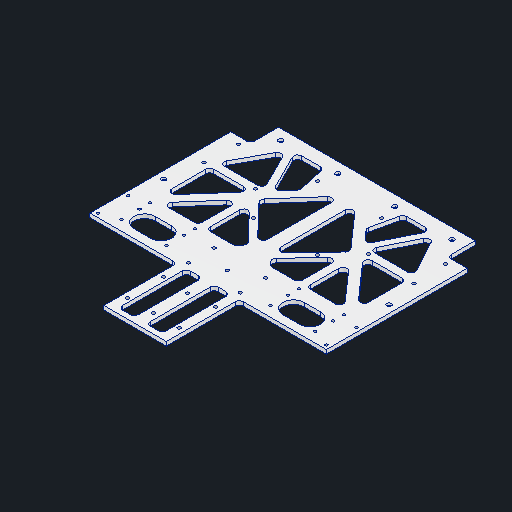
# Autodesk Inventor part: base
Saved by Autodesk Inventor 2023 (Build 270158000, 158)
## iProperties
Created: 2024-04-10
Part Number: base
Material: Aluminum 6061
Document SubType Name: Modeling
Designer: szymo
Density: 2.7 g/cm^3
Appearance: Aluminum - Flat
Mass: 125.073 g
Surface Area: 388.104 cm^2
Volume: 46.3232 cm^3
Author: szymo
Autodesk Inventor part; units mm, degrees
ref_plane "YZ Plane" through (0, 0, 0) normal (1, 0, 0) x (0, 1, 0)
ref_plane "XZ Plane" through (0, 0, 0) normal (0, 1, 0) x (-1, 0, 0)
ref_plane "XY Plane" through (0, 0, 0) normal (0, 0, 1) x (1, 0, 0)
sketch "Sketch2" plane through (0, 0, 0) normal (0, 1, 0) x (-1, 0, 0)
  line L0 (-89, 99) -> (89, 99)
  line L1 (89, 99) -> (89, -99)
  line L2 (89, -99) -> (-89, -99)
  line L3 (-89, -99) -> (-89, 99)
  line L4 (-89, 99) -> (89, -99) construction
  line L5 (89, 99) -> (-89, -99) construction
  line L6 (-89, 99) -> (89, 99)
  line L7 (89, 99) -> (89, -85)
  line L8 (89, -85) -> (-89, -85)
  line L9 (-89, -85) -> (-89, 99)
  line L10 (-4.5, 99) -> (-89, 99)
  line L11 (-89, 99) -> (-89, 42)
  line L12 (-89, 42) -> (-4.5, 42)
  line L13 (-4.5, 42) -> (-4.5, 99)
  line L14 (4.5, 99) -> (89, 99)
  line L15 (89, 99) -> (89, 42)
  line L16 (89, 42) -> (4.5, 42)
  line L17 (4.5, 42) -> (4.5, 99)
  line L18 (22.5, 77.5) -> (22.5, 66.5) projected
  line L19 (16.5, 66.5) -> (16.5, 77.5) projected
  line L20 (-22.5, 66.5) -> (-22.5, 77.5) projected
  line L21 (-16.5, 77.5) -> (-16.5, 66.5) projected
  line L22 (-23.5, 99) -> (-16.5, 99)
  line L23 (-16.5, 99) -> (-16.5, 42)
  line L24 (-16.5, 42) -> (-23.5, 42)
  line L25 (-23.5, 42) -> (-23.5, 99)
  line L26 (16.5, 99) -> (23.5, 99)
  line L27 (23.5, 99) -> (23.5, 42)
  line L28 (23.5, 42) -> (16.5, 42)
  line L29 (16.5, 42) -> (16.5, 99)
  line L30 (-89, 99) -> (89, 99)
  line L31 (89, 99) -> (89, 97)
  line L32 (89, 97) -> (-89, 97)
  line L33 (-89, 97) -> (-89, 99)
  line L34 (89, -85) -> (74, -85)
  line L35 (74, -85) -> (74, -64)
  line L36 (74, -64) -> (89, -64)
  line L37 (89, -64) -> (89, -85)
  line L38 (-89, -85) -> (-74, -85)
  line L39 (-74, -85) -> (-74, -64)
  line L40 (-74, -64) -> (-89, -64)
  line L41 (-89, -64) -> (-89, -85)
  line L42 (16.5, 97) -> (-16.5, 97)
  line L43 (-16.5, 97) -> (-16.5, 93)
  line L44 (-16.5, 93) -> (16.5, 93)
  line L45 (16.5, 93) -> (16.5, 97)
  line L46 (-84.4, -75) -> (-84.4, -71.5) projected
  line L47 (-84.4, -71.5) -> (-87, -71.5) projected
  line L48 (-87, -71.5) -> (-87, -75) projected
  line L49 (-87, -75) -> (-84.4, -75) projected
  line L50 (-79.6, -75) -> (-77, -75) projected
  line L51 (-77, -75) -> (-77, -71.5) projected
  line L52 (-77, -71.5) -> (-79.6, -71.5) projected
  line L53 (-79.6, -71.5) -> (-79.6, -75) projected
  line L54 (-75, -78) -> (-89, -78) projected
  line L55 (-89, -78) -> (-89, -63) projected
  line L56 (-89, -63) -> (-75, -63) projected
  line L57 (-75, -63) -> (-75, -78) projected
  circle A0 centre (-80.45, -67.25) radius 1.25 projected
  point P0 (0, 0)
  point P1 (4.5, 99)
  point P2 (-4.5, 99)
  point P3 (-89, 42)
  point P4 (89, 42)
  point P5 (4.5, 97)
  point P6 (-4.5, 97)
  point P7 (-16.5, 97)
  point P8 (-23.5, 97)
  point P9 (23.5, 97)
  point P10 (16.5, 98)
  point P11 (-4.5, 93)
  point P12 (4.5, 93)
  point P13 (16.5, 93)
  dimension "d8" = 178
  dimension "d9" = 198
  dimension "d10" = 14
  dimension "d11" = 84.5
  dimension "d13" = 84.5
  dimension "d17" = 9
  dimension "d18" = 2
  dimension "d19" = 15
  dimension "d20" = 21
  dimension "d21" = 15
  dimension "d22" = 21
  dimension "d75" = 55
  dimension "d76" = 55
  dimension "d77" = 7
  dimension "d78" = 7
  dimension "d79" = 4
  constraints: 84 end point, 20 parallel, 10 horizontal, 10 perpendicular, 10 point on line, 2 collinear, 2 midpoint, 5 other
  measures "d8" distance of L1.end L2.end
  measures "d9" distance of L0.end L1.end
  measures "d10" distance between parallel lines of L8 L2
  measures "d11" distance of L12.end L11.end
  measures "d13" distance of L15.end L16.end
  measures "d17" distance between parallel lines of L13 L17
  measures "d18" distance of L30.end L31.end
  measures "d19" distance of L35.end L36.end
  measures "d20" distance of L34.end L35.end
  measures "d21" distance of L40.end L39.end
  measures "d22" distance of L39.end L38.end
  measures "d75" distance between parallel lines of L32 L12
  measures "d76" distance between parallel lines of L32 L16
  measures "d77" distance between parallel lines of L23 L25
  measures "d78" distance between parallel lines of L27 L29
  measures "d79" distance of L43.end L42.end
extrude "Extrusion2" add sketch "Sketch2" along normal blind 3 contours L32 L23 L21 L12 L25 | L12 L13 L44 L17 L16 L1 L36 L35 L8 L39 L40 L57 L56 L3 | L32 L13 L44 L23 | L56 L57 L40 L3 | L32 L17 L44 L13 | L32 L29 L44 L17 | L32 L27 L16 L29 L19
fillet "Fillet5" radius 3 12 edges at (-16.5, 1.5, 42) (-4.5, 1.5, 42) (-23.5, 1.5, 42) (16.5, 1.5, 42) (-16.5, 1.5, 93) (-4.5, 1.5, 93) (4.5, 1.5, 93) (16.5, 1.5, 93) (4.5, 1.5, 42) (23.5, 1.5, 42) (74, 1.5, -64) (-74, 1.5, -64)
sketch "Sketch7" plane through (0, 3, 0) normal (0, 1, 0) x (1, 0, 0)
  circle A0 centre (78, 58.6725) radius 1.8 projected
  circle A1 centre (79, 33.8889) radius 1.8 projected
  circle A2 centre (42.4984, 36.1666) radius 1.8 projected
  circle A3 centre (24.1, 64.6) radius 1.6 projected
  circle A4 centre (24.1, 16.4) radius 1.6 projected
  circle A5 centre (-24.1, 16.4) radius 1.6 projected
  circle A6 centre (-24.1, 64.6) radius 1.6 projected
  circle A7 centre (-42.5, 36.1649) radius 1.8 projected
  circle A8 centre (-79, 33.8889) radius 1.8 projected
  circle A9 centre (-78, 58.6725) radius 1.8 projected
  circle A10 centre (19.5, -18.05) radius 1.8 projected
  circle A11 centre (19.5, -37.375) radius 1.8 projected
  circle A12 centre (19.5, -55.8) radius 1.8 projected
  circle A13 centre (19.4231, -83.3077) radius 1.8 projected
  circle A14 centre (0, -83.2) radius 1.8 projected
  circle A15 centre (-19.4231, -83.3077) radius 1.8 projected
  circle A16 centre (-19.5, -55.8) radius 1.8 projected
  circle A17 centre (0, -57.55) radius 1.8 projected
  circle A18 centre (0, -27.625) radius 1.8 projected
  circle A19 centre (-19.5, -37.375) radius 1.8 projected
  circle A20 centre (-19.5, -18.05) radius 1.8 projected
  point P0 (0, 0)
  point P1 (-19.5, -83.2)
  constraints: 20 coincident
hole "Hole3" at (19.4231, 3, 83.3077) at (0, 3, 83.2) at (-19.5, 3, 83.2) at (19.5, 3, 55.8) at (0, 3, 57.55) at (-19.5, 3, 55.8) at (-19.5, 3, 37.375) at (-19.5, 3, 18.05) at (0, 3, 27.625) at (19.5, 3, 37.375) at (19.5, 3, 18.05) at (79, 3, -33.8889) at (78, 3, -58.6725) at (42.4984, 3, -36.1666) at (24.1, 3, -16.4) at (-24.1, 3, -16.4) at (-24.1, 3, -64.6) at (24.1, 3, -64.6) at (-42.5, 3, -36.1649) at (-78, 3, -58.6725) at (-79, 3, -33.8889) direction (0, -1, 0) diameter 2.459 end through all thread size "M3x0.5" class "6H" standard "ISO Metric profile"
sketch "Sketch8" plane through (0, 3, 0) normal (0, 1, 0) x (1, 0, 0)
  circle A0 centre (72.95, -34.475) radius 1.45 projected
  circle A1 centre (72.95, -20.775) radius 1.45 projected
  circle A2 centre (39.125, -20.8375) radius 1.55 projected
  circle A3 centre (39.125, -34.4125) radius 1.55 projected
  circle A4 centre (-39.125, -20.8375) radius 1.55 projected
  circle A5 centre (-39.125, -34.4125) radius 1.55 projected
  circle A6 centre (-72.95, -34.475) radius 1.45 projected
  circle A7 centre (-72.95, -20.775) radius 1.45 projected
  circle A8 centre (86, -16.25) radius 2.3 projected
  circle A9 centre (86, -39) radius 2.3 projected
  circle A10 centre (86, 32.8889) radius 2.3 projected
  line L0 (89, -42) -> (83, -42) projected
  line L1 (89, 35.8889) -> (89, -42) projected
  line L2 (89, 35.8889) -> (83, 35.8889) projected
  line L3 (83, 29.8889) -> (83, 35.8889) projected
  line L4 (83, 29.8889) -> (87.4, 29.8889) projected
  line L5 (87.4, 29.8889) -> (87.4, 14.7889) projected
  line L6 (87.4, 14.7889) -> (79.4, 14.7889) projected
  line L7 (79.4, 2.7889) -> (79.4, 14.7889) projected
  line L8 (86, 2.7889) -> (79.4, 2.7889) projected
  line L9 (86, -13.25) -> (86, 2.7889) projected
  line L10 (86, -13.25) -> (83, -13.25) projected
  line L11 (83, -13.25) -> (83, -19.25) projected
  line L12 (83, -19.25) -> (86, -19.25) projected
  line L13 (86, -36) -> (86, -19.25) projected
  line L14 (86, -36) -> (83, -36) projected
  line L15 (83, -36) -> (83, -42) projected
  circle A11 centre (83.4, 10.7889) radius 2.6 projected
  circle A12 centre (-86, -39) radius 2.3 projected
  circle A13 centre (-86, -16.25) radius 2.3 projected
  line L16 (-86, -13.25) -> (-86, -0.1111) projected
  line L17 (-79.4, -0.1111) -> (-86, -0.1111) projected
  line L18 (-79.4, 11.8889) -> (-79.4, -0.1111) projected
  line L19 (-86, 11.8889) -> (-79.4, 11.8889) projected
  line L20 (-86, 11.8889) -> (-86, 29.8889) projected
  line L21 (-86, 29.8889) -> (-83, 29.8889) projected
  line L22 (-83, 29.8889) -> (-83, 35.8889) projected
  line L23 (-89, 35.8889) -> (-83, 35.8889) projected
  line L24 (-89, 35.8889) -> (-89, -42) projected
  line L25 (-89, -42) -> (-83, -42) projected
  line L26 (-83, -42) -> (-83, -36) projected
  line L27 (-83, -36) -> (-86, -36) projected
  line L28 (-86, -36) -> (-86, -19.25) projected
  line L29 (-86, -19.25) -> (-83, -19.25) projected
  line L30 (-83, -19.25) -> (-83, -13.25) projected
  line L31 (-83, -13.25) -> (-86, -13.25) projected
  circle A14 centre (-86, 32.8889) radius 2.3 projected
  circle A15 centre (-83.4, 7.8889) radius 2.6 projected
  line L32 (72.95, -34.475) -> (39.125, -12.8375)
  line L33 (72.95, -12.775) -> (39.125, -34.4125)
  line L34 (-39.125, -34.4125) -> (-72.95, -12.775)
  line L35 (-39.125, -12.8375) -> (-72.95, -34.4125)
  point P0 (0, 0)
  point P1 (56.0375, -23.5937)
  point P2 (-56.0375, -23.625)
  dimension "d90" = 8
  dimension "d91" = 8
  dimension "d92" = 8
  dimension "d93" = 8
  constraints: 12 coincident, 8 end point, 2 midpoint
  measures "d90" distance of A1.centre L33.start
  measures "d91" distance of L32.end A2.centre
  measures "d92" distance of point (-39.125, -20.837) L35.start
  measures "d93" distance of A7.centre L34.end
hole "Hole4" at (72.95, 3, 34.475) at (72.95, 3, 20.775) at (39.125, 3, 20.8375) at (39.125, 3, 34.4125) at (86, 3, 39) at (86, 3, 16.25) at (-86, 3, 39) at (-86, 3, 16.25) at (-72.95, 3, 20.775) at (-72.95, 3, 34.475) at (-39.125, 3, 34.4125) at (-39.125, 3, 20.8375) at (72.95, 3, 12.775) at (39.125, 3, 12.8375) at (-39.125, 3, 12.8375) at (-72.95, 3, 12.775) direction (0, -1, 0) diameter 2.013 end through all thread size "M2.5x0.45" class "6H" standard "ISO Metric profile"
sketch "Sketch9" plane through (0, 0, 0) normal (0, -1, 0) x (1, 0, 0)
  circle A0 centre (64.5, -77) radius 1.2295 projected
  circle A1 centre (21.5, -77) radius 1.2295 projected
  circle A2 centre (-21.5, -77) radius 1.2295 projected
  circle A3 centre (-64.5, -77) radius 1.2295 projected
  circle A4 centre (-83.4, -7.8889) radius 2.6 projected
  circle A5 centre (83.4, -10.7889) radius 2.6 projected
  point P0 (0, 0)
  constraints: 6 coincident
hole "Hole5" at (-83.4, 0, -7.8889) at (83.4, 0, -10.7889) at (64.5, 0, -77) at (21.5, 0, -77) at (-21.5, 0, -77) at (-64.5, 0, -77) direction (0, 1, 0) diameter 3.6 end through all countersink diameter 6.6 countersink angle 90 clearance for "Countersunk Flat Head Screw ISO 2009/7046" size "M3" standard "ISO"
sketch "Sketch11" plane through (0, 0, 0) normal (0, -1, 0) x (1, 0, 0)
  circle A0 centre (-21.5, -77) radius 3.3 projected
  circle A1 centre (64.5, -77) radius 3.3 projected
  circle A2 centre (-83.4, -7.8889) radius 3.3 projected
  circle A3 centre (83.4, -10.7889) radius 3.3 projected
  circle A4 centre (21.5, -77) radius 3.3 projected
  circle A5 centre (-64.5, -77) radius 3.3 projected
  circle A6 centre (-39.125, 12.8375) radius 1.0065 projected
  circle A7 centre (72.95, 12.775) radius 1.0065 projected
  circle A8 centre (-39.125, 34.4125) radius 1.0065 projected
  circle A9 centre (-72.95, 20.775) radius 1.0065 projected
  circle A10 centre (-86, 39) radius 1.0065 projected
  circle A11 centre (86, 39) radius 1.0065 projected
  circle A12 centre (39.125, 20.8375) radius 1.0065 projected
  circle A13 centre (72.95, 34.475) radius 1.0065 projected
  circle A14 centre (72.95, 20.775) radius 1.0065 projected
  circle A15 centre (39.125, 34.4125) radius 1.0065 projected
  circle A16 centre (86, 16.25) radius 1.0065 projected
  circle A17 centre (-86, 16.25) radius 1.0065 projected
  circle A18 centre (-72.95, 34.475) radius 1.0065 projected
  circle A19 centre (-39.125, 20.8375) radius 1.0065 projected
  circle A20 centre (39.125, 12.8375) radius 1.0065 projected
  circle A21 centre (-72.95, 12.775) radius 1.0065 projected
  circle A22 centre (-78, -58.6725) radius 1.2295 projected
  circle A23 centre (24.1, -64.6) radius 1.2295 projected
  circle A24 centre (-24.1, -16.4) radius 1.2295 projected
  circle A25 centre (42.4984, -36.1666) radius 1.2295 projected
  circle A26 centre (79, -33.8889) radius 1.2295 projected
  circle A27 centre (19.5, 37.375) radius 1.2295 projected
  circle A28 centre (-19.5, 18.05) radius 1.2295 projected
  circle A29 centre (-19.5, 55.8) radius 1.2295 projected
  circle A30 centre (19.5, 55.8) radius 1.2295 projected
  circle A31 centre (0, 83.2) radius 1.2295 projected
  circle A32 centre (19.4231, 83.3077) radius 1.2295 projected
  circle A33 centre (-19.5, 83.2) radius 1.2295 projected
  circle A34 centre (0, 57.55) radius 1.2295 projected
  circle A35 centre (-19.5, 37.375) radius 1.2295 projected
  circle A36 centre (0, 27.625) radius 1.2295 projected
  circle A37 centre (19.5, 18.05) radius 1.2295 projected
  circle A38 centre (78, -58.6725) radius 1.2295 projected
  circle A39 centre (24.1, -16.4) radius 1.2295 projected
  circle A40 centre (-24.1, -64.6) radius 1.2295 projected
  circle A41 centre (-42.5, -36.1649) radius 1.2295 projected
  circle A42 centre (-79, -33.8889) radius 1.2295 projected
  arc A43 (-13.5, 93) -> (-16.5, 90) centre (-13.5, 90) ccw projected
  line L0 (-7.5, 93) -> (-13.5, 93) projected
  arc A44 (-4.5, 90) -> (-7.5, 93) centre (-7.5, 90) ccw projected
  line L1 (-4.5, 45) -> (-4.5, 90) projected
  arc A45 (-7.5, 42) -> (-4.5, 45) centre (-7.5, 45) ccw projected
  line L2 (-13.5, 42) -> (-7.5, 42) projected
  arc A46 (-16.5, 45) -> (-13.5, 42) centre (-13.5, 45) ccw projected
  line L3 (-16.5, 90) -> (-16.5, 45) projected
  arc A47 (16.5, 90) -> (13.5, 93) centre (13.5, 90) ccw projected
  line L4 (16.5, 45) -> (16.5, 90) projected
  arc A48 (13.5, 42) -> (16.5, 45) centre (13.5, 45) ccw projected
  line L5 (7.5, 42) -> (13.5, 42) projected
  arc A49 (4.5, 45) -> (7.5, 42) centre (7.5, 45) ccw projected
  line L6 (4.5, 90) -> (4.5, 45) projected
  arc A50 (7.5, 93) -> (4.5, 90) centre (7.5, 90) ccw projected
  line L7 (13.5, 93) -> (7.5, 93) projected
  line L8 (-23.5, 97) -> (23.5, 97) projected
  line L9 (-23.5, 45) -> (-23.5, 97) projected
  arc A51 (-26.5, 42) -> (-23.5, 45) centre (-26.5, 45) ccw projected
  line L10 (-89, 42) -> (-26.5, 42) projected
  line L11 (-89, -64) -> (-89, 42) projected
  line L12 (-77, -64) -> (-89, -64) projected
  arc A52 (-74, -67) -> (-77, -64) centre (-77, -67) ccw projected
  line L13 (-74, -85) -> (-74, -67) projected
  line L14 (74, -85) -> (-74, -85) projected
  line L15 (74, -67) -> (74, -85) projected
  arc A53 (77, -64) -> (74, -67) centre (77, -67) ccw projected
  line L16 (89, -64) -> (77, -64) projected
  line L17 (89, 42) -> (89, -64) projected
  line L18 (26.5, 42) -> (89, 42) projected
  arc A54 (23.5, 45) -> (26.5, 42) centre (26.5, 45) ccw projected
  line L19 (23.5, 97) -> (23.5, 45) projected
  circle A55 centre (-42.5, -36.1649) radius 1.8 projected
  line L20 (-86, 0.1111) -> (-86, 42) projected
  line L21 (-89, 42) -> (-86, 42) projected
  line L22 (-89, 42) -> (-89, 38.75) projected
  line L23 (-89, 38.75) -> (-89, 13.5) projected
  line L24 (-89, 13.5) -> (-89, -81) projected
  line L25 (-89, -81) -> (-83, -81) projected
  line L26 (-83, -81) -> (-83, -75) projected
  line L27 (-83, -75) -> (-73, -75) projected
  line L28 (-73, -75) -> (-73, -53.3451) projected
  line L29 (-73, -53.3451) -> (-67, -53.3451) projected
  line L30 (-67, -53.3451) -> (-67, -42.9318) projected
  line L31 (-76.801, -42.9318) -> (-67, -42.9318) projected
  line L32 (-75, -34.8889) -> (-75, -29.8889) projected
  line L33 (-86, -29.8889) -> (-75, -29.8889) projected
  line L34 (-86, -29.8889) -> (-86, -11.8889) projected
  line L35 (-79.4, -11.8889) -> (-86, -11.8889) projected
  line L36 (-79.4, 0.1111) -> (-79.4, -11.8889) projected
  line L37 (-86, 0.1111) -> (-79.4, 0.1111) projected
  circle A56 centre (-83.5, -70.5) radius 1.75 projected
  circle A57 centre (-79, -33.8889) radius 1.8 projected
  circle A58 centre (-83.4, -7.8889) radius 2.6 projected
  circle A59 centre (-78, -58.6725) radius 1.8 projected
  circle A60 centre (78, -58.6725) radius 1.8 projected
  circle A61 centre (79, -33.8889) radius 1.8 projected
  circle A62 centre (83.4, -10.7889) radius 2.6 projected
  circle A63 centre (80.5, -70.5) radius 1.75 projected
  circle A64 centre (42.4984, -36.1666) radius 1.8 projected
  spline S0 degree 2 poles (89, 38.051) (88.5208, 39.25) (89, 40.449) knots 0 0 0 0.244949 0.244949 0.244949 weights 1 1.090909 1 projected
  line L38 (89, 42) -> (89, 40.449) projected
  line L39 (89, 42) -> (86, 42) projected
  line L40 (86, -2.7889) -> (86, 42) projected
  line L41 (79.4, -2.7889) -> (86, -2.7889) projected
  line L42 (79.4, -14.7889) -> (79.4, -2.7889) projected
  line L43 (86, -14.7889) -> (79.4, -14.7889) projected
  line L44 (86, -16.7889) -> (86, -14.7889) projected
  line L45 (86, -27.8889) -> (86, -16.7889) projected
  line L46 (86, -29.8889) -> (86, -27.8889) projected
  ellipse E0 centre (76.799, -27.2986) end of major axis (76.7969, -11.6653) minor radius 1.851 (76.801, -42.9318) -> (77.5308, -41.6649) ccw projected
  line L47 (76.801, -42.9318) -> (67, -42.9318) projected
  line L48 (67, -53.3451) -> (67, -42.9318) projected
  line L49 (73, -53.3451) -> (67, -53.3451) projected
  line L50 (73, -75) -> (73, -53.3451) projected
  line L51 (83, -75) -> (73, -75) projected
  line L52 (83, -81) -> (83, -75) projected
  line L53 (89, -81) -> (83, -81) projected
  line L54 (89, 14.801) -> (89, -81) projected
  spline S1 degree 2 poles (89, 14.801) (88.5208, 16) (89, 17.199) knots 0 0 0 0.244949 0.244949 0.244949 weights 1 1.090909 1 projected
  line L55 (89, 38.051) -> (89, 17.199) projected
  line L56 (27.5, -68) -> (27.5, -13) projected
  line L57 (27.5, -13) -> (-27.5, -13) projected
  line L58 (-27.5, -13) -> (-27.5, -68) projected
  line L59 (-27.5, -68) -> (27.5, -68) projected
  circle A65 centre (24.1, -64.6) radius 1.6 projected
  circle A66 centre (24.1, -16.4) radius 1.6 projected
  circle A67 centre (-24.1, -64.6) radius 1.6 projected
  circle A68 centre (-24.1, -16.4) radius 1.6 projected
  circle A69 centre (21.5, -77) radius 1.2295 projected
  circle A70 centre (-64.5, -77) radius 1.2295 projected
  circle A71 centre (-21.5, -77) radius 1.2295 projected
  circle A72 centre (64.5, -77) radius 1.2295 projected
  line L60 (-72, -70) -> (-72, -79) projected
  arc A73 (-74, -81) -> (-72, -79) centre (-74, -79) ccw projected
  line L61 (-74, -81) -> (-89, -81) projected
  line L62 (-89, -81) -> (-89, -85) projected
  line L63 (-89, -85) -> (89, -85) projected
  line L64 (89, -81) -> (89, -85) projected
  line L65 (89, -81) -> (74, -81) projected
  arc A74 (72, -79) -> (74, -81) centre (74, -79) ccw projected
  line L66 (72, -79) -> (72, -70) projected
  line L67 (57, -70) -> (72, -70) projected
  line L68 (57, -70) -> (57, -79) projected
  arc A75 (55, -81) -> (57, -79) centre (55, -79) ccw projected
  line L69 (55, -81) -> (31, -81) projected
  arc A76 (29, -79) -> (31, -81) centre (31, -79) ccw projected
  line L70 (29, -79) -> (29, -70) projected
  line L71 (14, -70) -> (29, -70) projected
  line L72 (14, -70) -> (14, -79) projected
  arc A77 (12, -81) -> (14, -79) centre (12, -79) ccw projected
  line L73 (12, -81) -> (-12, -81) projected
  arc A78 (-14, -79) -> (-12, -81) centre (-12, -79) ccw projected
  line L74 (-14, -79) -> (-14, -70) projected
  line L75 (-29, -70) -> (-14, -70) projected
  line L76 (-29, -70) -> (-29, -79) projected
  arc A79 (-31, -81) -> (-29, -79) centre (-31, -79) ccw projected
  line L77 (-31, -81) -> (-55, -81) projected
  arc A80 (-57, -79) -> (-55, -81) centre (-55, -79) ccw projected
  line L78 (-57, -79) -> (-57, -70) projected
  line L79 (-72, -70) -> (-57, -70) projected
  line L80 (-89, -85) -> (-89, -99) projected
  line L81 (-89, -99) -> (89, -99) projected
  line L82 (89, -85) -> (89, -99) projected
  line L83 (-89, -85) -> (89, -85) projected
  circle A81 centre (72.95, 34.475) radius 1.45 projected
  circle A82 centre (72.95, 20.775) radius 1.45 projected
  circle A83 centre (39.125, 34.4125) radius 1.55 projected
  circle A84 centre (39.125, 20.8375) radius 1.55 projected
  spline S2 degree 3 poles (65.7, 23.025) (65.7, 22.8819) (65.6837, 22.6312) (65.6334, 22.3458) (65.5819, 22.1333) (65.5405, 21.9923) (65.48, 21.8179) (65.4239, 21.6792) (65.3456, 21.5106) (65.2769, 21.3802) (65.184, 21.2227) (65.1043, 21.1011) (64.9982, 20.9549) (64.9083, 20.8425) (64.7662, 20.6811) (64.615, 20.5299) (64.3941, 20.3423) (64.2146, 20.2128) (64.0241, 20.0935) (63.8917, 20.0193) (63.7367, 19.9424) (63.63, 19.8951) (63.5206, 19.8513) (63.4473, 19.8241) (63.3368, 19.7865) (63.2255, 19.7528) (63.02, 19.6999) (62.7939, 19.6576) (62.4526, 19.6224) (62.1474, 19.6224) (61.8061, 19.6576) (61.58, 19.6999) (61.3745, 19.7528) (61.2632, 19.7865) (61.1527, 19.8241) (61.0794, 19.8513) (60.97, 19.8951) (60.8633, 19.9424) (60.7083, 20.0193) (60.5759, 20.0935) (60.3854, 20.2128) (60.2059, 20.3423) (59.985, 20.5299) (59.8338, 20.6811) (59.6917, 20.8425) (59.6018, 20.9549) (59.4957, 21.1011) (59.416, 21.2227) (59.3231, 21.3802) (59.2544, 21.5106) (59.1761, 21.6792) (59.12, 21.8179) (59.0595, 21.9923) (59.0181, 22.1333) (58.9666, 22.3458) (58.9163, 22.6312) (58.9, 22.8819) (58.9, 23.025) knots 0.368505 0.368505 0.368505 0.368505 0.400174 0.423925 0.431842 0.447677 0.455594 0.471428 0.479345 0.49518 0.503097 0.518931 0.526849 0.542683 0.5506 0.574352 0.590186 0.613938 0.621855 0.637689 0.645607 0.657482 0.661441 0.669358 0.673317 0.685193 0.69311 0.716861 0.732696 0.764365 0.780199 0.803951 0.811868 0.823744 0.827702 0.835619 0.839578 0.851454 0.859371 0.875205 0.883123 0.906874 0.922709 0.94646 0.954377 0.970212 0.978129 0.993963 1.00188 1.017715 1.025632 1.041466 1.049384 1.065218 1.073135 1.096887 1.128556 1.128556 1.128556 1.128556 projected
  line L84 (58.9, 23.025) -> (58.9, 32.225) projected
  spline S3 degree 3 poles (58.9, 32.225) (58.9, 32.3681) (58.9163, 32.6188) (58.9666, 32.9042) (59.0181, 33.1167) (59.0595, 33.2577) (59.12, 33.4321) (59.1761, 33.5708) (59.2544, 33.7394) (59.3231, 33.8698) (59.416, 34.0273) (59.4957, 34.1489) (59.6018, 34.2951) (59.6917, 34.4075) (59.8338, 34.5689) (59.985, 34.7201) (60.2059, 34.9077) (60.3854, 35.0372) (60.5759, 35.1565) (60.7083, 35.2307) (60.8633, 35.3076) (60.97, 35.3549) (61.0794, 35.3987) (61.1527, 35.4259) (61.2632, 35.4635) (61.3745, 35.4972) (61.58, 35.5501) (61.8061, 35.5924) (62.1474, 35.6276) (62.4526, 35.6276) (62.7939, 35.5924) (63.02, 35.5501) (63.2255, 35.4972) (63.3368, 35.4635) (63.4473, 35.4259) (63.5206, 35.3987) (63.63, 35.3549) (63.7367, 35.3076) (63.8917, 35.2307) (64.0241, 35.1565) (64.2146, 35.0372) (64.3941, 34.9077) (64.615, 34.7201) (64.7662, 34.5689) (64.9083, 34.4075) (64.9982, 34.2951) (65.1043, 34.1489) (65.184, 34.0273) (65.2769, 33.8698) (65.3456, 33.7394) (65.4239, 33.5708) (65.48, 33.4321) (65.5405, 33.2577) (65.5819, 33.1167) (65.6334, 32.9042) (65.6837, 32.6188) (65.7, 32.3681) (65.7, 32.225) knots -0.380025 -0.380025 -0.380025 -0.380025 -0.348357 -0.324605 -0.316688 -0.300853 -0.292936 -0.277102 -0.269185 -0.25335 -0.245433 -0.229599 -0.221682 -0.205847 -0.19793 -0.174178 -0.158344 -0.134592 -0.126675 -0.110841 -0.102924 -0.091048 -0.087089 -0.079172 -0.075213 -0.063338 -0.05542 -0.031669 -0.015834 0.015834 0.031669 0.05542 0.063338 0.075213 0.079172 0.087089 0.091048 0.102924 0.110841 0.126675 0.134592 0.158344 0.174178 0.19793 0.205847 0.221682 0.229599 0.245433 0.25335 0.269185 0.277102 0.292936 0.300853 0.316688 0.324605 0.348357 0.380025 0.380025 0.380025 0.380025 projected
  line L85 (65.7, 32.225) -> (65.7, 23.025) projected
  line L86 (27.2, 42) -> (86, 42) projected
  line L87 (27.2, 13.25) -> (27.2, 42) projected
  line L88 (27.2, 13.25) -> (86, 13.25) projected
  line L89 (86, 42) -> (86, 13.25) projected
  circle A85 centre (-72.95, 34.475) radius 1.45 projected
  circle A86 centre (-72.95, 20.775) radius 1.45 projected
  circle A87 centre (-39.125, 34.4125) radius 1.55 projected
  circle A88 centre (-39.125, 20.8375) radius 1.55 projected
  spline S4 degree 3 poles (-65.7, 23.025) (-65.7, 22.8819) (-65.6837, 22.6312) (-65.6334, 22.3458) (-65.5819, 22.1333) (-65.5405, 21.9923) (-65.48, 21.8179) (-65.4239, 21.6792) (-65.3456, 21.5106) (-65.2769, 21.3802) (-65.184, 21.2227) (-65.1043, 21.1011) (-64.9982, 20.9549) (-64.9083, 20.8425) (-64.7662, 20.6811) (-64.615, 20.5299) (-64.3941, 20.3423) (-64.2146, 20.2128) (-64.0241, 20.0935) (-63.8917, 20.0193) (-63.7367, 19.9424) (-63.63, 19.8951) (-63.5206, 19.8513) (-63.4473, 19.8241) (-63.3368, 19.7865) (-63.2255, 19.7528) (-63.02, 19.6999) (-62.7939, 19.6576) (-62.4526, 19.6224) (-62.1474, 19.6224) (-61.8061, 19.6576) (-61.58, 19.6999) (-61.3745, 19.7528) (-61.2632, 19.7865) (-61.1527, 19.8241) (-61.0794, 19.8513) (-60.97, 19.8951) (-60.8633, 19.9424) (-60.7083, 20.0193) (-60.5759, 20.0935) (-60.3854, 20.2128) (-60.2059, 20.3423) (-59.985, 20.5299) (-59.8338, 20.6811) (-59.6917, 20.8425) (-59.6018, 20.9549) (-59.4957, 21.1011) (-59.416, 21.2227) (-59.3231, 21.3802) (-59.2544, 21.5106) (-59.1761, 21.6792) (-59.12, 21.8179) (-59.0595, 21.9923) (-59.0181, 22.1333) (-58.9666, 22.3458) (-58.9163, 22.6312) (-58.9, 22.8819) (-58.9, 23.025) knots 0.368505 0.368505 0.368505 0.368505 0.400174 0.423925 0.431842 0.447677 0.455594 0.471428 0.479345 0.49518 0.503097 0.518931 0.526849 0.542683 0.5506 0.574352 0.590186 0.613938 0.621855 0.637689 0.645607 0.657482 0.661441 0.669358 0.673317 0.685193 0.69311 0.716861 0.732696 0.764365 0.780199 0.803951 0.811868 0.823744 0.827702 0.835619 0.839578 0.851454 0.859371 0.875205 0.883123 0.906874 0.922709 0.94646 0.954377 0.970212 0.978129 0.993963 1.00188 1.017715 1.025632 1.041466 1.049384 1.065218 1.073135 1.096887 1.128556 1.128556 1.128556 1.128556 projected
  line L90 (-65.7, 32.225) -> (-65.7, 23.025) projected
  spline S5 degree 3 poles (-58.9, 32.225) (-58.9, 32.3681) (-58.9163, 32.6188) (-58.9666, 32.9042) (-59.0181, 33.1167) (-59.0595, 33.2577) (-59.12, 33.4321) (-59.1761, 33.5708) (-59.2544, 33.7394) (-59.3231, 33.8698) (-59.416, 34.0273) (-59.4957, 34.1489) (-59.6018, 34.2951) (-59.6917, 34.4075) (-59.8338, 34.5689) (-59.985, 34.7201) (-60.2059, 34.9077) (-60.3854, 35.0372) (-60.5759, 35.1565) (-60.7083, 35.2307) (-60.8633, 35.3076) (-60.97, 35.3549) (-61.0794, 35.3987) (-61.1527, 35.4259) (-61.2632, 35.4635) (-61.3745, 35.4972) (-61.58, 35.5501) (-61.8061, 35.5924) (-62.1474, 35.6276) (-62.4526, 35.6276) (-62.7939, 35.5924) (-63.02, 35.5501) (-63.2255, 35.4972) (-63.3368, 35.4635) (-63.4473, 35.4259) (-63.5206, 35.3987) (-63.63, 35.3549) (-63.7367, 35.3076) (-63.8917, 35.2307) (-64.0241, 35.1565) (-64.2146, 35.0372) (-64.3941, 34.9077) (-64.615, 34.7201) (-64.7662, 34.5689) (-64.9083, 34.4075) (-64.9982, 34.2951) (-65.1043, 34.1489) (-65.184, 34.0273) (-65.2769, 33.8698) (-65.3456, 33.7394) (-65.4239, 33.5708) (-65.48, 33.4321) (-65.5405, 33.2577) (-65.5819, 33.1167) (-65.6334, 32.9042) (-65.6837, 32.6188) (-65.7, 32.3681) (-65.7, 32.225) knots -0.380025 -0.380025 -0.380025 -0.380025 -0.348357 -0.324605 -0.316688 -0.300853 -0.292936 -0.277102 -0.269185 -0.25335 -0.245433 -0.229599 -0.221682 -0.205847 -0.19793 -0.174178 -0.158344 -0.134592 -0.126675 -0.110841 -0.102924 -0.091048 -0.087089 -0.079172 -0.075213 -0.063338 -0.05542 -0.031669 -0.015834 0.015834 0.031669 0.05542 0.063338 0.075213 0.079172 0.087089 0.091048 0.102924 0.110841 0.126675 0.134592 0.158344 0.174178 0.19793 0.205847 0.221682 0.229599 0.245433 0.25335 0.269185 0.277102 0.292936 0.300853 0.316688 0.324605 0.348357 0.380025 0.380025 0.380025 0.380025 projected
  line L91 (-58.9, 23.025) -> (-58.9, 32.225) projected
  line L92 (-27.2, 42) -> (-86, 42) projected
  line L93 (-86, 42) -> (-86, 13.25) projected
  line L94 (-27.2, 13.25) -> (-86, 13.25) projected
  line L95 (-27.2, 13.25) -> (-27.2, 42) projected
  line L96 (-22.5, 14.25) -> (22.5, 14.25) projected
  line L97 (22.5, 14.25) -> (22.5, 13.25) projected
  line L98 (-22.5, 13.25) -> (22.5, 13.25) projected
  line L99 (-22.5, 14.25) -> (-22.5, 13.25) projected
  line L100 (-27.2, 13.25) -> (-27.2, 42) projected
  line L101 (-27.2, 13.25) -> (-22.7, 13.25) projected
  line L102 (-22.7, 13.25) -> (-22.7, 42) projected
  line L103 (-27.2, 42) -> (-22.7, 42) projected
  line L104 (27.2, 13.25) -> (27.2, 42) projected
  line L105 (27.2, 42) -> (22.7, 42) projected
  line L106 (22.7, 13.25) -> (22.7, 42) projected
  line L107 (27.2, 13.25) -> (22.7, 13.25) projected
  line L108 (-77.0142, -3.75) -> (-9.0142, -3.75) projected
  line L109 (-9.0142, -3.75) -> (-9.0142, 11.25) projected
  line L110 (-9.0142, 11.25) -> (-77.0142, 11.25) projected
  line L111 (-77.0142, 11.25) -> (-77.0142, -3.75) projected
  line L112 (77.6433, -8.75) -> (11.6433, -8.75) projected
  line L113 (77.6433, 11.25) -> (77.6433, -8.75) projected
  line L114 (11.6433, 11.25) -> (77.6433, 11.25) projected
  line L115 (11.6433, -8.75) -> (11.6433, 11.25) projected
  line L116 (-74, -85) -> (74, -85)
  line L117 (74, -85) -> (74, -70)
  line L118 (-74, -70) -> (-74, -85)
  line L119 (-89, -64) -> (-74, -64)
  line L120 (-74, -64) -> (-74, 42)
  line L121 (-74, 42) -> (-89, 42)
  line L122 (-89, 42) -> (-89, -64)
  line L123 (89, 42) -> (89, -64) projected
  line L124 (89, -64) -> (74, -64)
  line L125 (74, -64) -> (74, 42)
  line L126 (74, 42) -> (89, 42)
  line L127 (89, 42) -> (89, -64)
  line L128 (-74, 8.7685) -> (74, 8.7685)
  circle A89 centre (-72.95, 12.775) radius 1.0065 projected
  line L129 (0, -75) -> (-74, 8.7685) construction
  line L130 (0, -75) -> (74, 8.7685) construction
  line L131 (-4.6701, -75) -> (-74, 3.4819)
  line L132 (4.6701, -75) -> (74, 3.4819)
  line L133 (0, -69.7134) -> (74, 14.0551)
  line L134 (0, -69.7134) -> (-74, 14.0551)
  line L135 (0, 8.7685) -> (-36.0614, -28.8917) construction
  line L136 (0, 8.7685) -> (36.0614, -28.8917) construction
  line L137 (-3.4613, 8.7685) -> (-37.7223, -27.0115)
  line L138 (-34.4005, -30.7719) -> (0, 5.1537)
  line L139 (0, 5.1537) -> (34.4005, -30.7719)
  line L140 (37.7223, -27.0115) -> (3.4613, 8.7685)
  line L141 (-74, -39.1649) -> (-36.3263, -39.1649)
  line L142 (36.3263, -39.1649) -> (74, -39.1649)
  line L143 (-40.7223, -23.6155) -> (-40.7223, 8.7685)
  line L144 (-34.7223, -23.8785) -> (-34.7223, 8.7685)
  line L145 (34.7223, -23.8785) -> (34.7223, 8.7685)
  line L146 (40.7223, -23.6155) -> (40.7223, 8.7685)
  line L147 (-37.7223, -27.0115) -> (-37.7223, 8.7685) construction
  line L148 (37.7223, -27.0115) -> (37.7223, 8.7685) construction
  line L149 (0, 5.1537) -> (0, -69.7134) construction
  line L150 (5, -64.0534) -> (5, -0.0679)
  line L151 (-5, -0.0679) -> (-5, -64.0534)
  line L152 (-5, -0.0679) -> (-13.8364, 8.7685)
  line L153 (5, -0.0679) -> (13.8364, 8.7685)
  line L154 (-57, -75) -> (57, -75)
  line L155 (-30.121, -75) -> (-24.9693, -52.0212)
  line L156 (30.121, -75) -> (24.9693, -52.0212)
  line L157 (-54.2434, -75) -> (-74, -39.1649)
  line L158 (54.2434, -75) -> (74, -39.1649)
  line L159 (-74, -33.1649) -> (-41.6266, -33.1649)
  line L160 (74, -33.1649) -> (41.6266, -33.1649)
  circle A90 centre (-42.5, -36.1649) radius 1.2295 projected
  line L161 (-42.5, -36.1649) -> (-74, -36.1649) construction
  line L162 (74, -36.1666) -> (42.4984, -36.1666) construction
  line L163 (-86, 27.625) -> (-22.7, 27.625)
  circle A91 centre (-62.3, 27.625) radius 8
  circle A92 centre (-49.775, 27.625) radius 8
  line L164 (-62.3, 35.625) -> (-49.775, 35.625)
  line L165 (-49.775, 19.625) -> (-62.3, 19.625)
  line L166 (0, 57.55) -> (0, 27.625) construction
  line L167 (27.2, 27.625) -> (86, 27.625)
  circle A93 centre (62.3, 27.625) radius 8
  circle A94 centre (49.775, 27.625) radius 8
  line L168 (62.3, 35.625) -> (49.775, 35.625)
  line L169 (49.775, 19.625) -> (62.3, 19.625)
  line L170 (-54.2434, -75) -> (-36.3263, -39.1649) construction
  line L171 (54.2434, -75) -> (36.3263, -39.1649) construction
  line L172 (51.4483, -75) -> (34.5414, -41.1854)
  line L173 (55.7092, -72.3413) -> (39.1214, -39.1649)
  line L174 (-34.5414, -41.1854) -> (-51.4483, -75)
  line L175 (-39.1214, -39.1649) -> (-55.7092, -72.3413)
  point P0 (-72.95, 11.7685)
  point P1 (24.3056, -13)
  point P2 (27.5, -16.336)
  point P3 (-27.5, -16.336)
  point P4 (-24.3056, -13)
  point P5 (-9.0142, 2.9694)
  point P6 (-9.0142, 8.7685)
  point P7 (-8.5364, 3.4684)
  point P8 (11.6433, 8.7685)
  point P9 (11.6433, 6.5754)
  point P10 (8.5364, 3.4684)
  point P11 (74, -42.9318)
  point P12 (67, -51.8617)
  point P13 (71.9233, -42.9318)
  point P14 (-74, -42.9318)
  point P15 (-71.9233, -42.9318)
  point P16 (-67, -51.8617)
  point P17 (27.5, -49.1564)
  point P18 (27.5, -63.3093)
  point P19 (-27.5, -63.3093)
  point P20 (-27.5, -49.1564)
  point P21 (69.3299, 8.7685)
  point P22 (-69.3299, 8.7685)
  point P23 (-86, 17.2565)
  point P24 (-86, 15.2435)
  point P25 (-86, 40.0065)
  point P26 (-86, 37.9935)
  point P27 (-74, 33.475)
  point P28 (-74, 35.475)
  point P29 (-74, 19.775)
  point P30 (-74, 21.775)
  point P31 (86, 37.9935)
  point P32 (86, 40.0065)
  point P33 (86, 15.2435)
  point P34 (86, 17.2565)
  point P35 (74, 21.775)
  point P36 (74, 19.775)
  point P37 (74, 35.475)
  point P38 (74, 33.475)
  point P39 (10.8538, -68)
  point P40 (-10.8538, -68)
  point P41 (24.1249, -75)
  point P42 (18.8751, -75)
  point P43 (-27.5, -38.5833)
  point P44 (-1.5136, -68)
  point P45 (1.5136, -68)
  point P46 (27.5, -38.5833)
  point P47 (-24.1249, -75)
  point P48 (-18.8751, -75)
  point P49 (5, -13)
  point P50 (27.5, -23.5655)
  point P51 (17.383, -13)
  point P52 (-5, -13)
  point P53 (-17.383, -13)
  point P54 (-27.5, -23.5655)
  dimension "d146" = 15
  dimension "d147" = 15
  dimension "d150" = 3
  dimension "d151" = 3.5
  dimension "d152" = 7
  dimension "d153" = 7
  dimension "d154" = 3.5
  dimension "d155" = 5
  dimension "d156" = 2.5
  dimension "d157" = 5
  dimension "d158" = 2.5
  dimension "d159" = 3
  dimension "d160" = 6
  dimension "d161" = 6
  dimension "d162" = 3
  dimension "d167" = 5
  dimension "d169" = 10
  dimension "d170" = 45
  dimension "d171" = 45
  dimension "d172" = 3.2
  dimension "d175" = 3.6
  dimension "d176" = 3.2
  dimension "d177" = 3.6
  dimension "d178" = 3
  dimension "d179" = 6
  dimension "d180" = 6
  dimension "d181" = 2.9984
  dimension "d182" = 10
  dimension "d183" = 14.375
  dimension "d184" = 14.375
  dimension "d185" = 3.4
  dimension "d186" = 3.4
  dimension "d188" = 10.65
  dimension "d189" = 10.65
  dimension "d190" = 3.4
  dimension "d191" = 3.4
  dimension "d192" = 10.65
  dimension "d193" = 10.65
  dimension "d199" = 5
  dimension "d200" = 2.5
  dimension "d202" = 5
  dimension "d203" = 2.5
  constraints: 114 end point, 55 point on line, 23 parallel, 8 point on circle, 7 vertical, 5 horizontal, 5 perpendicular, 4 centre point, 4 midpoint, 4 tangent, 2 equal radius, 1 vertical alignment, 36 other
  measures "d146" distance of L121.end L120.end
  measures "d147" distance of L125.end L126.end
  measures "d151" distance between parallel lines of L129 L131
  measures "d152" distance between parallel lines of L131 L134
  measures "d153" distance between parallel lines of L133 L132
  measures "d154" distance between parallel lines of L130 L132
  measures "d155" distance between parallel lines of L137 L138
  measures "d156" distance between parallel lines of L138 L135
  measures "d157" distance between parallel lines of L140 L139
  measures "d158" distance between parallel lines of L136 L140
  measures "d159" distance between parallel lines of L147 L144
  measures "d160" distance between parallel lines of L143 L144
  measures "d161" distance between parallel lines of L145 L146
  measures "d162" distance between parallel lines of L148 L146
  measures "d167" distance between parallel lines of L149 L150
  measures "d169" distance between parallel lines of L151 L150
  measures "d170" angle to the sketch x axis of L152
  measures "d171" angle to the sketch x axis of L153
  measures "d172" diameter of A67
  measures "d175" distance from line of L155 A40.centre
  measures "d176" diameter of A65
  measures "d177" distance from line of L156 A23.centre
  measures "d178" distance between parallel lines of L161 L141
  measures "d179" distance between parallel lines of L159 L141
  measures "d180" distance between parallel lines of L160 L142
  measures "d181" distance between parallel lines of L162 L142
  measures "d183" distance between parallel lines of L92 L163
  measures "d184" distance between parallel lines of L163 L94
  measures "d185" distance from line of A91.centre L91
  measures "d186" distance from line of L90 A91.centre
  measures "d188" horizontal distance of A9.centre A91.centre
  measures "d189" horizontal distance of A92.centre A19.centre
  measures "d190" distance from line of L85 A93.centre
  measures "d191" distance from line of L84 A93.centre
  measures "d192" horizontal distance of A93.centre A14.centre
  measures "d193" horizontal distance of A12.centre A94.centre
  measures "d199" distance between parallel lines of L172 L173
  measures "d200" distance between parallel lines of L171 L173
  measures "d202" distance between parallel lines of L175 L174
  measures "d203" distance between parallel lines of L170 L174
extrude "Extrusion5" cut sketch "Sketch11" against normal up to next contours L155 L154 L174 L131 L58 | L58 L131 L155 | L134 L58 L138 L57 L151 | L132 L56 L156 | L134 L138 L58 | L157 L30 L31 L141 L175 | L150 L57 L139 L56 L133 | L57 L138 L151 | L56 L132 L172 L154 L156 | L159 L120 L108 L131 | L56 L139 L133 | L150 L139 L115 L112 L57 | L137 L144 L108 L57 L58 | L58 L57 L137 | L157 L31 L30 | L108 L120 L131 | L137 L109 L152 | L134 L108 L143 | L134 L128 L143 L108 | L140 L57 L56 | L56 L57 L140 L112 L145 | L112 L115 L139 | L153 L115 L140 | L108 L144 L128 L152 L109 L137 | L132 L112 L125 L160 | L142 L158 L47 L48 L173 | L146 L112 L133 | L140 L115 L153 L128 L145 L112 | L132 L125 L112 | L112 L146 L128 L133 | L158 L48 L47 | L20 A17 | A10 L20 | A91 S5 L90 L163 | L163 L90 S4 A91 | L163 L91 S4 L90 | L90 S5 L91 L163 | A91 A92 L163 L91 S5 | L164 A92 A91 | S4 L91 L163 A92 A91 | A91 A92 L165 | A92 A91 L163 | L163 A91 A92 | A91 L163 A92 | A92 L163 A91 | A93 S2 L85 L167 | L167 L85 S3 A93 | A94 A93 L167 | L167 A93 A94 | L167 L84 S3 L85 | L85 S2 L84 L167 | S3 L84 L167 A94 A93 | A93 A94 L168 | A93 A94 L167 L84 S2 | L169 A94 A93 | A93 A94 L167 | L167 A94 A93 picked at (-85.6977, 16.3956) picked at (-85.6977, 39.1456)
fillet "Fillet8" radius 3 40 edges at (-30.121, 1.5, -75) (-74, 1.5, -39.1649) (-24.9693, 1.5, -52.0212) (24.9693, 1.5, -52.0212) (74, 1.5, -39.1649) (30.121, 1.5, -75) (41.6266, 1.5, -33.1649) (74, 1.5, -33.1649) (74, 1.5, 3.4819) (-74, 1.5, 3.4819) (-41.6266, 1.5, -33.1649) (-74, 1.5, -33.1649) (-69.3299, 1.5, 8.7685) (-40.7223, 1.5, 8.7685) (-40.7223, 1.5, -23.6155) (-34.7223, 1.5, -23.8785) (-34.7223, 1.5, 8.7685) (-13.8364, 1.5, 8.7685) (-8.5364, 1.5, 3.4684) (8.5364, 1.5, 3.4684) (13.8364, 1.5, 8.7685) (34.7223, 1.5, 8.7685) (34.7223, 1.5, -23.8785) (40.7223, 1.5, -23.6155) (40.7223, 1.5, 8.7685) (69.3299, 1.5, 8.7685) (34.4005, 1.5, -30.7719) (5, 1.5, -64.0534) (-5, 1.5, -64.0534) (-34.4005, 1.5, -30.7719) (-5, 1.5, -0.0679) (5, 1.5, -0.0679) (-55.7092, 1.5, -72.3413) (-51.4483, 1.5, -75) (-34.5414, 1.5, -41.1854) (-39.1214, 1.5, -39.1649) (51.4483, 1.5, -75) (55.7092, 1.5, -72.3413) (39.1214, 1.5, -39.1649) (34.5414, 1.5, -41.1854)
equation "\"d11\" = d13"
body "Solid2"
